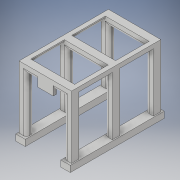
# Autodesk Inventor part: gris
Saved by Autodesk Inventor 2018 (Build 220112000, 112)
## iProperties
Created: 2021-02-15
Part Number: gris
Material: Generic
Document SubType Name: Modeling
Designer: Joel Olguin Lopez
Density: 1 g/cm^3
Appearance: Default
Author: Joel Olguin Lopez
Autodesk Inventor part; units mm, degrees
ref_plane "YZ Plane" through (0, 0, 0) normal (1, 0, 0) x (0, 1, 0)
ref_plane "XZ Plane" through (0, 0, 0) normal (0, 1, 0) x (-1, 0, 0)
ref_plane "XY Plane" through (0, 0, 0) normal (0, 0, 1) x (1, 0, 0)
sketch "Boceto1" plane through (0, 0, 0) normal (0, 0, 1) x (1, 0, 0)
  line L0 (19.05, -12.7) -> (-19.05, -12.7)
  line L1 (-19.05, -12.7) -> (-19.05, 12.7)
  line L2 (-19.05, 12.7) -> (19.05, 12.7)
  line L3 (19.05, 12.7) -> (19.05, -12.7)
  line L4 (19.05, -12.7) -> (-19.05, 12.7) construction
  line L5 (-19.05, -12.7) -> (19.05, 12.7) construction
  line L6 (163.83, -12.7) -> (201.93, -12.7)
  line L7 (201.93, -12.7) -> (201.93, 12.7)
  line L8 (201.93, 12.7) -> (163.83, 12.7)
  line L9 (163.83, 12.7) -> (163.83, -12.7)
  line L10 (163.83, -12.7) -> (201.93, 12.7) construction
  line L11 (201.93, -12.7) -> (163.83, 12.7) construction
  point P0 (0, 0)
  point P1 (182.88, 0)
  point P2 (182.88, 0)
  point P3 (0, 0)
  dimension "d0" = 38.1
  dimension "d1" = 25.4
  dimension "d27" = 38.1
  dimension "d28" = 25.4
  dimension "d29" = 182.88
  constraints: 24 end point, 6 midpoint, 4 parallel, 2 horizontal, 2 perpendicular, 1 horizontal alignment
  measures "d0" distance of L1.end L2.end
  measures "d1" distance of L2.end L0.start
  measures "d27" distance of L7.end L8.end
  measures "d28" distance of L6.end L7.end
  measures "d29" distance of point (182.88, 0) point (0, 0)
extrude "Extrusión1" add sketch "Boceto1" along normal mid plane 381
sketch "Boceto2" plane through (-19.05, 12.7, 190.5) normal (0, 1, 0) x (1, 0, 0)
  line L0 (34.1004, 371.7805) -> (3.9996, 371.7805)
  line L1 (3.9996, 371.7805) -> (3.9996, 341.6815)
  line L2 (3.9996, 341.6815) -> (34.1004, 341.6815)
  line L3 (34.1004, 341.6815) -> (34.1004, 371.7805)
  line L4 (34.1004, 371.7805) -> (3.9996, 341.6815) construction
  line L5 (3.9996, 371.7805) -> (34.1004, 341.6815) construction
  line L6 (34.1004, 205.5495) -> (3.9996, 205.5495)
  line L7 (3.9996, 205.5495) -> (3.9996, 175.4505)
  line L8 (3.9996, 175.4505) -> (34.1004, 175.4505)
  line L9 (34.1004, 175.4505) -> (34.1004, 205.5495)
  line L10 (34.1004, 205.5495) -> (3.9996, 175.4505) construction
  line L11 (3.9996, 205.5495) -> (34.1004, 175.4505) construction
  line L12 (34.1004, 39.3065) -> (3.9996, 39.3065)
  line L13 (3.9996, 39.3065) -> (3.9996, 9.2075)
  line L14 (3.9996, 9.2075) -> (34.1004, 9.2075)
  line L15 (34.1004, 9.2075) -> (34.1004, 39.3065)
  line L16 (34.1004, 39.3065) -> (3.9996, 9.2075) construction
  line L17 (3.9996, 39.3065) -> (34.1004, 9.2075) construction
  line L18 (38.1, 0) -> (0, 0) projected
  line L19 (0, 0) -> (0, 381) projected
  point P0 (19.05, 190.5)
  point P1 (19.05, 356.731)
  point P2 (19.05, 24.257)
  dimension "d4" = 30.1007
  dimension "d5" = 30.099
  dimension "d6" = 356.731
  dimension "d7" = 19.05
  dimension "d8" = 30.099
  dimension "d9" = 30.099
  dimension "d10" = 24.257
  dimension "d11" = 30.1007
  constraints: 36 end point, 6 midpoint, 6 parallel, 3 horizontal, 3 perpendicular, 2 point on line
  measures "d4" distance of L1.end L2.end
  measures "d5" distance of L0.end L1.end
  measures "d6" distance from line of L18 point (19.05, 356.731)
  measures "d7" distance from line of L19 point (19.05, 356.731)
  measures "d8" distance of L6.end L7.end
  measures "d9" distance of L12.end L13.end
  measures "d10" distance from line of L18 point (19.05, 24.257)
  measures "d11" distance of L12.start L12.end
extrude "Extrusión2" add sketch "Boceto2" along normal blind 254
sketch "Boceto3" plane through (15.0504, 12.7, 181.2925) normal (1, 0, 0) x (0, 0, -1)
  line L0 (0, 0) -> (0, 254) projected
  line L1 (30.099, 254) -> (0, 254)
  line L2 (0, 254) -> (0, 223.901)
  line L3 (0, 223.901) -> (30.099, 223.901)
  line L4 (30.099, 223.901) -> (30.099, 254)
  line L5 (166.243, 0) -> (166.243, 254) projected
  line L6 (196.342, 254) -> (166.243, 254)
  line L7 (166.243, 254) -> (166.243, 223.901)
  line L8 (166.243, 223.901) -> (196.342, 223.901)
  line L9 (196.342, 223.901) -> (196.342, 254)
  line L10 (332.474, 0) -> (332.474, 254) projected
  line L11 (362.573, 254) -> (332.474, 254)
  line L12 (332.474, 254) -> (332.474, 223.901)
  line L13 (332.474, 223.901) -> (362.573, 223.901)
  line L14 (362.573, 223.901) -> (362.573, 254)
  point P0 (181.2925, -12.7)
  dimension "d14" = 30.099
  dimension "d15" = 30.099
  dimension "d16" = 30.099
  constraints: 24 end point, 6 parallel, 3 horizontal, 3 perpendicular, 3 point on line
  measures "d14" distance of L3.end L1.start
  measures "d15" distance of L8.end L6.start
  measures "d16" distance of L13.end L11.start
extrude "Extrusión3" add sketch "Boceto3" along normal blind 152.4
sketch "Boceto4" plane through (-19.05, 266.7, 190.5) normal (0, 1, 0) x (1, 0, 0)
  line L0 (186.5004, 371.7805) -> (186.5004, 341.6815) projected
  line L1 (186.5004, 341.6815) -> (216.5994, 341.6815)
  line L2 (216.5994, 341.6815) -> (216.5994, 371.7805)
  line L3 (216.5994, 371.7805) -> (186.5004, 371.7805)
  line L4 (186.5004, 371.7805) -> (186.5004, 341.6815)
  line L5 (186.5004, 175.4505) -> (186.5004, 205.5495) projected
  line L6 (186.5004, 175.4505) -> (216.5994, 175.4505)
  line L7 (216.5994, 175.4505) -> (216.5994, 205.5495)
  line L8 (216.5994, 205.5495) -> (186.5004, 205.5495)
  line L9 (186.5004, 205.5495) -> (186.5004, 175.4505)
  line L10 (186.5004, 9.2075) -> (186.5004, 39.3065) projected
  line L11 (186.5004, 9.2075) -> (216.5994, 9.2075)
  line L12 (216.5994, 9.2075) -> (216.5994, 39.3065)
  line L13 (216.5994, 39.3065) -> (186.5004, 39.3065)
  line L14 (186.5004, 39.3065) -> (186.5004, 9.2075)
  point P0 (19.05, 190.5)
  dimension "d19" = 30.099
  dimension "d20" = 30.099
  dimension "d21" = 30.099
  dimension "d22" = 30.099
  dimension "d23" = 30.099
  dimension "d24" = 30.099
  constraints: 24 end point, 6 parallel, 3 horizontal, 3 perpendicular
  measures "d19" distance of L2.end L3.end
  measures "d20" distance of L1.end L2.end
  measures "d21" distance of L7.end L8.end
  measures "d22" distance of L6.end L7.end
  measures "d23" distance of L12.end L13.end
  measures "d24" distance of L11.end L12.end
extrude "Extrusión4" add sketch "Boceto4" against normal blind 254
sketch "Boceto5" plane through (-15.0504, 12.7, 181.2925) normal (0, 0, 1) x (1, 0, 0)
  line L0 (30.1007, 223.901) -> (182.5007, 223.901) projected
  line L1 (138.9293, 223.901) -> (75.6023, 223.901)
  line L2 (75.6023, 223.901) -> (75.6023, 199.8624)
  line L3 (75.6023, 199.8624) -> (138.9293, 199.8624)
  line L4 (138.9293, 199.8624) -> (138.9293, 223.901)
  line L5 (0, 0) -> (0, 254) projected
  point P0 (15.0504, -12.7)
  dimension "d30" = 24.0386
  dimension "d31" = 63.327
  dimension "d32" = 138.9293
  constraints: 8 end point, 2 parallel, 1 horizontal, 1 perpendicular, 1 point on line
  measures "d30" distance of L3.end L1.start
  measures "d31" distance of L2.end L3.end
  measures "d32" distance between parallel lines of L5 L4
extrude "Extrusión5" add sketch "Boceto5" against normal blind 12.7
fillet "Empalme1" radius 12.7 19 edges at (91.2504, 236.601, -181.2805) (15.0504, 124.6505, -181.2805) (167.4504, 124.6505, -181.2805) (167.4504, 124.6505, -151.1815) (91.2504, 236.601, -151.1815) (91.2504, 236.601, -15.0495) (15.0504, 124.6505, -15.0495) (91.2504, 236.601, 15.0495) (167.4504, 124.6505, 15.0495) (15.0504, 124.6505, -151.1815) (167.4504, 124.6505, 181.2925) (167.4504, 124.6505, 151.1935) (145.6646, 236.601, 181.2925) (37.8011, 236.601, 181.2925) (15.0504, 124.6505, 181.2925) (91.2504, 236.601, 151.1935) (15.0504, 124.6505, 151.1935) (167.4504, 124.6505, -15.0495) (15.0504, 124.6505, 15.0495)
sketch "Boceto6" plane through (-15.0504, 12.7, 15.0495) normal (0, 0, 1) x (1, 0, 0)
  line L0 (212.5997, 254) -> (212.5997, 0) projected
  line L1 (195.2007, 236.601) -> (182.5007, 223.901) projected
  line L2 (212.5997, 254) -> (195.2007, 254)
  line L3 (195.2007, 254) -> (195.2007, 236.601)
  line L4 (195.2007, 236.601) -> (212.5997, 236.601)
  line L5 (212.5997, 236.601) -> (212.5997, 254)
  line L6 (0, 254) -> (212.5997, 254) projected
  line L7 (30.1007, 223.901) -> (17.4007, 236.601) projected
  line L8 (0, 254) -> (17.4007, 254)
  line L9 (17.4007, 254) -> (17.4007, 236.601)
  line L10 (17.4007, 236.601) -> (0, 236.601)
  line L11 (0, 236.601) -> (0, 254)
  point P0 (15.0504, -12.7)
  constraints: 16 end point, 4 parallel, 2 horizontal, 2 perpendicular
extrude "Extrusión6" add sketch "Boceto6" along normal up to next
sketch "Boceto7" plane through (-15.0504, 12.7, -15.0495) normal (0, 0, -1) x (-1, 0, 0)
  line L0 (0, 254) -> (-212.5997, 254) projected
  line L1 (-17.4007, 236.601) -> (-195.2007, 236.601) projected
  line L2 (0, 254) -> (-17.4007, 254)
  line L3 (-17.4007, 254) -> (-17.4007, 236.601)
  line L4 (-17.4007, 236.601) -> (0, 236.601)
  line L5 (0, 236.601) -> (0, 254)
  line L6 (-212.5997, 254) -> (-212.5997, 0) projected
  line L7 (-195.2007, 236.601) -> (-195.2007, 0) projected
  line L8 (-212.5997, 254) -> (-195.2007, 254)
  line L9 (-195.2007, 254) -> (-195.2007, 236.601)
  line L10 (-195.2007, 236.601) -> (-212.5997, 236.601)
  line L11 (-212.5997, 236.601) -> (-212.5997, 254)
  point P0 (-15.0504, -12.7)
  constraints: 16 end point, 4 parallel, 2 horizontal, 2 perpendicular
extrude "Extrusión7" add sketch "Boceto7" along normal up to next contours L5 L4 L3 L0 | L9 L10 L6 L0
fillet "Empalme2" radius 12.7 4 edges at (2.3504, 249.301, 83.1215) (2.3504, 249.301, -83.1155) (180.1504, 249.301, 83.1215) (180.1504, 249.301, -83.1155)
